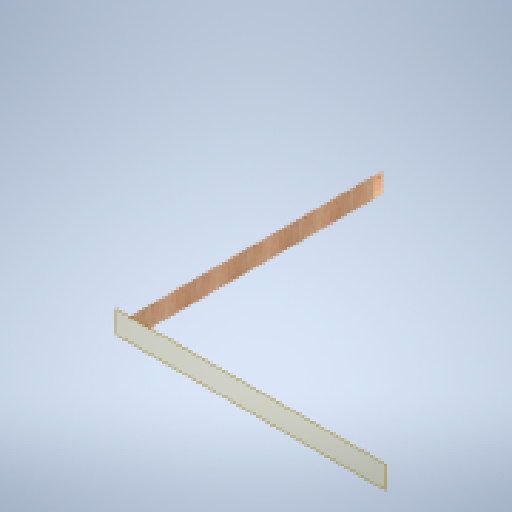
# Autodesk Inventor part: Leg slant.2
Saved by Autodesk Inventor 2025 (Build 290162000, 162)
## iProperties
Created: 2024-09-05
Part Number: Leg slant.2
Material: Wood (Birch)
Document SubType Name: Modeling
Designer: Win
Density: 0.55 g/cm^3
Appearance: Birch - Natural Polished
Author: Win
Autodesk Inventor part; units mm, degrees
ref_plane "YZ Plane" through (0, 0, 0) normal (1, 0, 0) x (0, 1, 0)
ref_plane "XZ Plane" through (0, 0, 0) normal (0, 1, 0) x (-1, 0, 0)
ref_plane "XY Plane" through (0, 0, 0) normal (0, 0, 1) x (1, 0, 0)
ref_plane "Work Plane1" through (-365.1942, 0, 0) normal (0, 0, 1) x (1, 0, 0)
sketch "Sketch1" plane through (-365.1942, 0, 0) normal (0, 0, 1) x (1, 0, 0)
  line L0 (365.2323, -2653.287) -> (365.2323, -2551.687) projected
  line L1 (365.2323, -2551.687) -> (-853.9677, -2551.687) projected
  line L2 (-853.9677, -2551.687) -> (-853.9677, -2653.287) projected
  line L3 (-853.9677, -2653.287) -> (365.2323, -2653.287) projected
  line L4 (365.2323, -2551.687) -> (416.0323, -2551.687) projected
  line L5 (416.0323, -1332.487) -> (416.0323, -2551.687) projected
  line L6 (365.2323, -1332.487) -> (416.0323, -1332.487) projected
  line L7 (365.2323, -1332.487) -> (365.2323, -2551.687) projected
  line L8 (365.2323, -1332.487) -> (365.2323, -1434.087)
  line L9 (-853.9677, -2551.687) -> (-752.3677, -2551.687)
  line L10 (-752.3677, -2551.687) -> (365.2323, -1434.087)
  line L11 (365.2323, -1332.487) -> (-853.9677, -2551.687)
  point P0 (365.1942, 0)
  dimension "d0" = 101.6
  dimension "d1" = 101.6
  constraints: 8 end point, 2 point on line, 1 other
  measures "d0" distance of L6.start L8.end
  measures "d1" distance of L1.end L9.end
extrude "Extrusion1" add sketch "Sketch1" against normal blind 50.8 contours L1 L11 L7 L10
body "Solid1"
